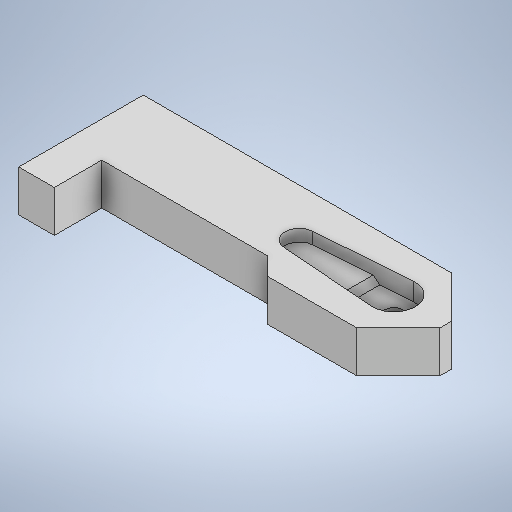
# Autodesk Inventor part: GrabberArmV2
Saved by Autodesk Inventor 2025.1 (Build 291241000, 241)
## iProperties
Created: 2025-02-23
Part Number: GrabberArmV2
Material: Generic
Document SubType Name: Modeling
Designer: 13156
Density: 1 g/cm^3
Appearance: Default
Author: 13156
Autodesk Inventor part; units mm, degrees
ref_plane "YZ Plane" through (0, 0, 0) normal (1, 0, 0) x (0, 1, 0)
ref_plane "XZ Plane" through (0, 0, 0) normal (0, 1, 0) x (-1, 0, 0)
ref_plane "XY Plane" through (0, 0, 0) normal (0, 0, 1) x (1, 0, 0)
sketch "Sketch1" plane through (0, 0, 0) normal (0, 1, 0) x (-1, 0, 0)
  circle A0 centre (0, 0) radius 3.6
  line L0 (0, 0) -> (15.95, 0) construction
  circle A1 centre (15.95, 0) radius 2.4
  line L1 (0.2708, 3.5898) -> (16.1306, 2.3932)
  line L2 (0.2708, -3.5898) -> (16.1306, -2.3932)
  line L3 (5.6, 3.1877) -> (5.6, -3.1877)
  line L4 (0, 0) -> (-3.6, 0)
  circle A2 centre (0, 0) radius 1.55
  circle A3 centre (15.95, 0) radius 0.85
  circle A4 centre (0, 0) radius 2.975
  line L5 (0, 0) -> (14.0413, 0)
  line L6 (0, 0) -> (0, -12.0932)
  line L7 (0, -17.1119) -> (0, 18.0186) projected
  line L8 (-8.75, 8) -> (-8.75, -8)
  line L9 (50.25, -8) -> (50.25, 13)
  line L10 (50.25, 13) -> (44.25, 13)
  line L11 (44.25, 13) -> (44.25, 5)
  line L12 (-8.75, 8) -> (-2.975, 8)
  line L13 (-2.975, 8) -> (16.25, 8)
  line L14 (16.25, 8) -> (16.25, 5)
  line L15 (16.25, 5) -> (44.25, 5)
  line L16 (50.25, -8) -> (-8.75, -8)
  point P0 (47.25, 13)
  dimension "d14" = 7.2
  dimension "d15" = 4.8
  dimension "d16" = 15.95
  dimension "d17" = 9.2
  dimension "d18" = 3.1
  dimension "d19" = 1.7
  dimension "d20" = 5.95
  dimension "d21" = 0
  dimension "d25" = 8.75
  dimension "d27" = 6
  dimension "d42" = 59
  dimension "d43" = 13
  dimension "d46" = 25
  dimension "d47" = 8
  dimension "d48" = 8
  constraints: 33 end point, 5 centre point, 5 perpendicular, 5 point on circle, 4 coincident, 4 tangent, 4 vertical, 3 horizontal, 3 point on line, 1 collinear, 1 midpoint, 1 other
  measures "d14" diameter of A0
  measures "d15" diameter of A1
  measures "d16" distance of L0.end point (0, 0)
  measures "d17" distance from line of L4.end L3
  measures "d18" diameter of A2
  measures "d19" diameter of A3
  measures "d20" diameter of A4
  measures "d21" distance from line of L7 L0.start
  measures "d25" distance from line of point (0, 0) L8
  measures "d27" distance of L9.end L10.end
  measures "d42" distance of L9.start L8.end
  measures "d43" distance between parallel lines of L15 L16
  measures "d46" distance from line of L14.end L8
  measures "d47" distance from line of L15 point (47.25, 13)
  measures "d48" distance from line of point (0, 0) L16
extrude "Extrusion1" add sketch "Sketch1" against normal blind 7 contours L5 A4 L7 A0 | L5 L3 L2 A0 | A0 L6 A4 L5 | A0 L1 L3 L5 | A0 L7 L13 L14 L15 L11 L10 L9 L16 L6 L2 A1 L1 | L5 A2 L7 A4 | A4 L6 A2 L5 | L5 A1 L2 L3 | L3 L1 A1 L5 | L7 A4 L4 A0 | A0 L6 L16 L8 L12 L13 L7 | A0 L4 A4 L6 | L7 A2 L4 A4 | A4 L4 A2 L6 | A1 | A3
extrude "Extrusion2" cut sketch "Sketch1" against normal blind 2 contours L5 A4 L7 A0 | L5 L3 L2 A0 | A0 L6 A4 L5 | A0 L1 L3 L5 | L5 A2 L7 A4 | A4 L6 A2 L5 | L5 A1 L2 L3 | L3 L1 A1 L5 | L7 A4 L4 A0 | A0 L4 A4 L6 | L7 A2 L4 A4 | A4 L4 A2 L6 | L5 L7 A2 | A2 L6 L5 | A1 | L7 L4 A2 | A2 L4 L6 | A3
extrude "Extrusion3" cut sketch "Sketch1" against normal blind 3 contours L5 A4 L7 A0 | L5 L3 L2 A0 | A0 L6 A4 L5 | A0 L1 L3 L5 | L5 A2 L7 A4 | A4 L6 A2 L5 | L7 A4 L4 A0 | A0 L4 A4 L6 | L7 A2 L4 A4 | A4 L4 A2 L6
chamfer "Chamfer1" distance 1 angle 45 1 edges at (-5.6, -2, 0)
chamfer "Chamfer3" distance 3 angle 45 1 edges at (-16.25, -3.5, 8)
chamfer "Chamfer5" distance 7 angle 45 2 edges at (8.75, -3.5, 8) (8.75, -3.5, -8)
body "Solid1"
